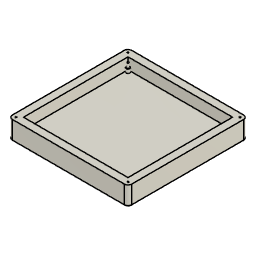
CAD (Autodesk Fusion 360 design; units mm, degrees)
Autodesk Fusion 360 part; units mm, degrees
sketch "Sketch1" plane through (0, 0, 0) normal (0, 0, 1) x (1, 0, 0)
  line L0 (80, 80) -> (-80, 80)
  line L1 (-80, 80) -> (-80, -80)
  line L2 (-80, -80) -> (80, -80)
  line L3 (80, -80) -> (80, 80)
  line L4 (80, 80) -> (-80, -80) construction
  line L5 (-80, 80) -> (80, -80) construction
  dimension "d3" = 160
  dimension "d4" = 160
  constraint horizontal L0
  constraint perpendicular L0 L1
  constraint parallel L0 L2
  constraint parallel L1 L3
  constraint coincident L4 origin
  constraint coincident L5 origin
  measures "d3" distance of L1.end L2.end
  measures "d4" distance of L0.end L1.end
extrude "Extrude1" add sketch "Sketch1" along normal blind 30 makes body 1
ref_plane "WorkPlane1" through (0, 0, 25) normal (0, 0, 1) x (1, 0, 0)
split "Split1" by plane through (0, 0, 25) normal (0, 0, 1) bodies 1 makes body 2 at (-26.6667, 26.6667, 30)
shell "Shell1" thickness 10 removed faces 1 at (26.6667, -26.6667, 25) on bodies 1
fillet "Fillet1" radius 5 8 edges at (80, 80, 12.5) (-80, -80, 12.5) (80, -80, 12.5) (-80, 80, 12.5) (80, 80, 27.5) (-80, -80, 27.5) (80, -80, 27.5) (-80, 80, 27.5) on bodies 1 2
fillet "Fillet2" radius 1 16 edges at (-80, 0, 0) (-78.5355, -78.5355, 0) (0, -80, 0) (78.5355, -78.5355, 0) (80, 0, 0) (78.5355, 78.5355, 0) (0, 80, 0) (-78.5355, 78.5355, 0) (80, 0, 30) (78.5355, -78.5355, 30) (0, -80, 30) (-78.5355, -78.5355, 30) (-80, 0, 30) (-78.5355, 78.5355, 30) (0, 80, 30) (78.5355, 78.5355, 30) on bodies 1 2
hole "Hole1" at (-75, 75, 30) direction (0, 0, -1) diameter 2.076 depth 20 tip angle 118 bodies 1 2
thread "Thread1" "ISO Metric profile 2.5 M2.5x0.45 6H" thread offset 0 thread depth 15
hole "Hole2" at (75, 75, 30) direction (0, 0, -1) diameter 2.076 depth 20 tip angle 118 bodies 1 2
thread "Thread2" "ISO Metric profile 2.5 M2.5x0.45 6H" thread offset 0 thread depth 15
hole "Hole3" at (75, -75, 30) direction (0, 0, -1) diameter 2.076 depth 20 tip angle 118 bodies 1 2
thread "Thread3" "ISO Metric profile 2.5 M2.5x0.45 6H" thread offset 0 thread depth 15
hole "Hole4" at (-75, -75, 30) direction (0, 0, -1) diameter 2.076 depth 20 tip angle 118 bodies 1 2
thread "Thread4" "ISO Metric profile 2.5 M2.5x0.45 6H" thread offset 0 thread depth 15
sketch "Sketch2" plane through (0, 0, 10) normal (0, 0, 1) x (-1, 0, 0)
  line L0 (70, -70) -> (70, 70)
  line L1 (70, 70) -> (-70, 70)
  line L2 (-70, 70) -> (-70, -70)
  line L3 (-70, -70) -> (70, -70)
  circle A0 centre (67.5, -67.5) radius 2.5
  circle A1 centre (-67.5, -67.5) radius 2.5
  circle A2 centre (-67.5, 67.5) radius 2.5
  circle A3 centre (67.5, 67.5) radius 2.5
  dimension "d33" = 5
  dimension "d34" = 5
  dimension "d35" = 5
  dimension "d36" = 5
  constraint tangent L3 A0
  constraint tangent L0 A0
  constraint tangent L3 A1
  constraint tangent L2 A1
  constraint tangent L1 A2
  constraint tangent L2 A2
  constraint tangent L1 A3
  constraint tangent L0 A3
  measures "d33" diameter of A0
  measures "d34" diameter of A1
  measures "d35" diameter of A2
  measures "d36" diameter of A3
extrude "Extrude2" add sketch "Sketch2" along normal blind 5 separate body contours A0 | A3 | A1 | A2 makes body 3 at (69.8492, -68.3551, 13.3333) makes body 4 at (69.8492, 66.6449, 13.3333) makes body 5 at (-65.1508, -68.3551, 13.3333) makes body 6 at (-65.1508, 66.6449, 13.3333)
cylinder "CylinderPrimitive1" add diameter 2.5 height 5 placed x (1, 0, 0) y (0, 1, 0) z (0, 0, 1) at (-67.5, -67.5, 15) bodies 5
cylinder "CylinderPrimitive2" add diameter 2.5 height 6 placed x (1, 0, 0) y (0, 1, 0) z (0, 0, 1) at (-67.5, 67.5, 15) bodies 6
cylinder "CylinderPrimitive3" add diameter 2.5 height 5 placed x (1, 0, 0) y (0, 1, 0) z (0, 0, 1) at (67.5, 67.5, 15) bodies 4
cylinder "CylinderPrimitive4" add diameter 2.5 height 5 placed x (1, 0, 0) y (0, 1, 0) z (0, 0, 1) at (67.5, -67.5, 15) bodies 3
hidden bodies 2
equation "width = 160 mm"
equation "height = 30 mm"
equation "d3 = width"
equation "d4 = width"
equation "d5 = height"
named bodies: "Bottom", "Top"
